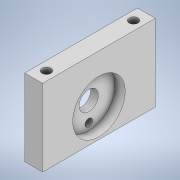
# Autodesk Inventor part: motor_front
Saved by Autodesk Inventor 2020 (Build 240168000, 168)
## iProperties
Created: 2023-11-06
Part Number: motor_front
Material: Типовые
Document SubType Name: Modeling
Designer: denis
Density: 1 g/cm^3
Appearance: По умолчанию
Author: denis
Autodesk Inventor part; units mm, degrees
ref_plane "YZ Plane" through (0, 0, 0) normal (1, 0, 0) x (0, 1, 0)
ref_plane "XZ Plane" through (0, 0, 0) normal (0, 1, 0) x (-1, 0, 0)
ref_plane "XY Plane" through (0, 0, 0) normal (0, 0, 1) x (1, 0, 0)
sketch "Эскиз1" plane through (0, 0, 0) normal (0, 1, 0) x (-1, 0, 0)
  line L0 (7, 44) -> (0, 44)
  line L1 (0, 44) -> (0, 0)
  line L2 (0, 0) -> (7, 0)
  line L3 (7, 0) -> (7, 44)
  line L4 (-16.3445, 0) -> (14.925, 0) construction
  line L5 (0, 24.3748) -> (0, -24.0504) construction
  circle A0 centre (3.5, 39) radius 1.75
  line L6 (3.5, 44) -> (3.5, 0) construction
  line L7 (7, 22) -> (0, 22) construction
  circle A1 centre (3.5, 5) radius 1.75
  point P0 (0, 0)
  dimension "d0" = 44
  dimension "d1" = 7
  dimension "d2" = 3.5
  dimension "d5" = 34
  constraints: 16 end point, 3 horizontal, 3 perpendicular, 3 point on line, 2 centre point, 2 collinear, 2 midpoint, 2 parallel, 2 vertical, 1 symmetric about line, 1 other
  measures "d0" distance of L2.end L0.start
  measures "d1" distance of L0.start L0.end
  measures "d2" diameter of A0
  measures "d5" distance of A1.centre A0.centre
extrude "Выдавливание1" add sketch "Эскиз1" along normal blind 30
sketch "Эскиз2" plane through (0, 0, 44) normal (1, 0, 0) x (0, 0, -1)
  line L0 (0, 0) -> (44, 0) construction
  line L1 (44, 0) -> (44, 30) construction
  line L2 (0, 30) -> (44, 30) construction
  line L3 (0, 0) -> (0, 30) construction
  line L4 (44, 30) -> (0, 30) construction
  line L5 (22, 30) -> (22, 0) construction
  line L6 (44, 0) -> (0, 0) construction
  line L7 (0, 0) -> (0, 30) construction
  line L8 (0, 15) -> (44, 15) construction
  line L9 (44, 0) -> (44, 30) construction
  circle A0 centre (22, 11.2) radius 10.25
  circle A1 centre (22, 11.2) radius 3.75
  circle A2 centre (22, 18.7) radius 1.5
  line L10 (18.25, 11.2) -> (25.75, 11.2) construction
  circle A3 centre (22, 3.7) radius 1.5
  dimension "d8" = 20.5
  dimension "d9" = 11.2
  dimension "d10" = 7.5
  dimension "d11" = 3
  dimension "d12" = 15
  constraints: 6 end point, 5 midpoint, 4 centre point, 2 point on circle, 2 point on line, 1 coincident, 1 horizontal, 1 symmetric about line, 1 other
  measures "d8" diameter of A0
  measures "d9" distance from line of L0 A0.centre
  measures "d10" diameter of A1
  measures "d11" diameter of A2
  measures "d12" distance of A3.centre A2.centre
extrude "Выдавливание2" cut sketch "Эскиз2" against normal blind 30 contours A1 | A2 | A3
extrude "Выдавливание3" cut sketch "Эскиз2" against normal blind 4
